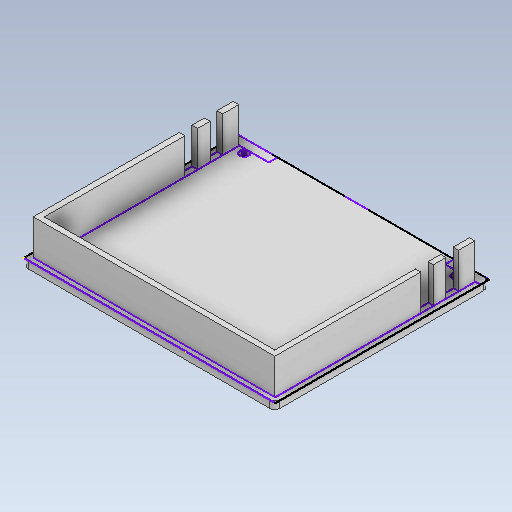
# Autodesk Inventor part: Part2
Saved by Autodesk Inventor 2020.2 (Build 242310000, 310)
## iProperties
Created: 2019-12-02
Part Number: Part2
Material: Generic
Document SubType Name: Modeling
Designer: athiy
Density: 1 g/cm^3
Appearance: Default
Author: athiy
Autodesk Inventor part; units mm, degrees
ref_plane "YZ Plane" through (0, 0, 0) normal (1, 0, 0) x (0, 1, 0)
ref_plane "XZ Plane" through (0, 0, 0) normal (0, 1, 0) x (-1, 0, 0)
ref_plane "XY Plane" through (0, 0, 0) normal (0, 0, 1) x (1, 0, 0)
sketch "Sketch1" plane through (0, 0, 0) normal (0, 1, 0) x (-1, 0, 0)
  line L0 (0, 0) -> (100, 0)
  line L1 (100, 0) -> (100, -85)
  line L2 (100, -85) -> (0, -85)
  line L3 (0, -85) -> (0, 0)
  line L4 (100, -85) -> (100, -81.5)
  line L5 (100, -85) -> (0, -85)
  line L6 (0, 0) -> (100, 0)
  dimension "d0" = 100
  dimension "d1" = 85
  constraints: 14 end point, 4 equal length, 1 horizontal, 1 perpendicular, 1 point on line
  measures "d0" distance of L1.end L2.end
  measures "d1" distance of L0.end L1.end
extrude "Extrusion1" add sketch "Sketch1" along normal blind 3
sketch "Sketch5" plane through (0, 3, 0) normal (0, 1, 0) x (1, 0, 0)
  line L0 (-100, 85.001914) -> (0, 85.001914)
  line L1 (0, 85.001914) -> (0, 0.001914)
  line L2 (0, 0.001914) -> (-100, 0.001914)
  line L3 (0, 0.001914) -> (0, 3.501877)
  line L4 (0, 0.001914) -> (-100, 0.001914)
  line L5 (-100, 85.001914) -> (0, 85.001914)
  line L6 (-100, 85) -> (-100, 0)
  line L7 (-100, 85) -> (-100, 0)
  line L8 (0, 81.501879) -> (-13.977379, 81.501879)
  line L9 (0, 85) -> (-100, 85)
  line L10 (-13.977379, 81.501879) -> (-13.977379, 85)
  line L11 (0, 0) -> (0, 85)
  line L12 (0, 81.501879) -> (0, 85)
  line L13 (0, 85) -> (-13.977379, 85)
  line L14 (0, 81.501879) -> (-6, 81.501879)
  line L15 (-100, 85) -> (-100, 0)
  line L16 (-100, 0) -> (0, 0)
  line L17 (-100, 81.501917) -> (-84.168275, 81.501917)
  line L18 (-84.168275, 85) -> (-84.168275, 81.501917)
  line L19 (-93.931804, 81.467894) -> (-95.682804, 81.467894)
  line L20 (-98.248671, 81.501917) -> (-100, 81.501917)
  line L21 (-47.950989, 85) -> (-11.964435, 85)
  line L22 (-57.205258, 85) -> (-86.408023, 85)
  circle A0 centre (-7.75, 7.751877) radius 1.75
  circle A1 centre (-92.181804, 7.751877) radius 1.75
  circle A2 centre (-7.724421, 79.777458) radius 1.724421
  circle A3 centre (-92.171647, 79.74176) radius 1.760157
  line L23 (-6, 6.035046) -> (-6, 6.001877)
  line L24 (-1.751121, 81.501879) -> (-1.951121, 81.501879)
  line L25 (-1.951121, 81.501879) -> (-1.951121, 1.951914)
  line L26 (-98.048671, 1.951914) -> (-98.048671, 81.501917)
  line L27 (-98.048671, 1.951914) -> (-1.951121, 1.951914)
  line L28 (-4.180804, 81.501879) -> (-4.080804, 81.501879)
  line L29 (-4.080804, 81.501879) -> (-4.080804, 4.116343)
  line L30 (-95.682804, 81.501917) -> (-95.782804, 81.501917)
  line L31 (-95.782804, 81.501917) -> (-95.782804, 4.116343)
  line L32 (-95.782804, 4.116343) -> (-4.080804, 4.116343)
  line L33 (0, 85) -> (0, 75)
  line L34 (-1.951121, 75) -> (-4.080804, 75)
  line L35 (-4.080804, 75) -> (-4.080804, 70)
  line L36 (-4.080804, 70) -> (-1.951121, 70)
  line L37 (-1.951121, 70) -> (-1.951121, 65)
  line L38 (-1.951121, 65) -> (-4.080804, 65)
  line L39 (-4.080804, 65) -> (-4.080804, 60)
  line L40 (-4.080804, 60) -> (-1.951121, 60)
  line L41 (-95.782804, 60) -> (-98.048671, 60)
  line L42 (-95.782804, 65) -> (-98.048671, 65)
  line L43 (-95.782804, 70) -> (-98.048671, 70)
  line L44 (-95.782804, 75) -> (-98.048671, 75)
  point P0 (-92.171647, 81.501917)
  point P1 (-7.724421, 81.501879)
  dimension "d22" = 100
  dimension "d23" = 85
  dimension "d61" = 3.5
  dimension "d74" = 0.1
  constraints: 82 end point, 32 point on line, 17 perpendicular, 5 horizontal, 4 centre point, 4 collinear, 3 tangent, 2 parallel
  measures "d22" distance of L1.end L2.end
  measures "d23" distance of L0.end L1.end
  measures "d61" diameter of A0
  measures "d74" distance of L30.start L30.end
extrude "Extrusion10" add sketch "Sketch5" along normal blind 14 contours L17 L31 L44 L26 | L43 L31 L42 L26 | L41 L31 L32 L29 L40 L25 L27 L26 | L25 L34 L29 L8 | L25 L38 L29 L36
extrude "Extrusion11" cut sketch "Sketch5" against normal through all contours A3 | A2 | A0 | A1
fillet "Fillet1" radius 2 4 edges at (-100, 1.5, -85) (-100, 1.5, 0) (0, 1.5, -85) (0, 1.5, 0)
body "Solid1"
